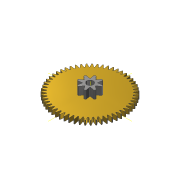
# Autodesk Inventor part: empty
Saved by Autodesk Inventor 2014 (Build 180170000, 170)
## iProperties
Created: 2015-04-13
Part Number: empty
Material: Generic
Document SubType Name: Modeling
Designer: Martin
Density: 1 g/cm^3
Appearance: Default
Author: Martin
Autodesk Inventor part; units mm, degrees
ref_plane "YZ Plane" through (0, 0, 0) normal (1, 0, 0) x (0, 1, 0)
ref_plane "XZ Plane" through (0, 0, 0) normal (0, 1, 0) x (-1, 0, 0)
ref_plane "XY Plane" through (0, 0, 0) normal (0, 0, 1) x (1, 0, 0)
sketch "Sketch1" plane through (0, 0, 0) normal (1, 0, 0) x (0, 1, 0)
  line L0 (0, -22.56081) -> (0, 23.084566)
  line L1 (-1.56, 0) -> (9.36, 0)
  line L2 (0, 16.563798) -> (0, -16.040042)
  line L3 (0.75, 0) -> (0.75, 2.8)
  line L4 (0.75, 2.8) -> (2.125, 2.8)
  line L5 (2.125, 2.8) -> (2.125, 1)
  line L6 (2.125, 1) -> (7.8, 1)
  line L7 (7.8, 1) -> (7.8, 0)
  line L8 (0.75, 0) -> (7.8, 0)
  point P0 (0, 0)
  dimension "d0" = 15.6
  dimension "d1" = 1
  dimension "d2" = 2.8
  dimension "d3" = 4.25
  dimension "d5" = 1.5
  constraints: 14 end point, 4 parallel, 4 point on line, 1 collinear, 1 perpendicular
  measures "d0" diameter of L7 L2
  measures "d1" distance of L6.end L7.end
  measures "d2" distance between parallel lines of L1 L4
  measures "d3" diameter of L5 L2
  measures "d5" diameter of L3 L2
sketch "Sketch1 outline for Revolution1" plane through (0, 0, 0) normal (1, 0, 0) x (0, 1, 0)
  line L0 (0.75, 2.8) -> (0.75, 0)
  line L1 (2.125, 2.8) -> (0.75, 2.8)
  line L2 (2.125, 1) -> (2.125, 2.8)
  line L3 (7.8, 1) -> (2.125, 1)
  line L4 (7.8, 0) -> (7.8, 1)
  line L5 (0.75, 0) -> (7.8, 0)
revolve "Revolution1" add sketch "Sketch1 outline for Revolution1" angle 360 about axis through (0, 0, 16.563798) along (0, 0, -1)
sketch "Sketch2" plane through (0, 0, 1) normal (0, 0, 1) x (1, 0, 0)
  circle A0 centre (0, 0) radius 2.125
  line L0 (0, -10.921041) -> (0, 10.926244)
  line L1 (0, 2.125) -> (0.44563, 7.78726) construction
  line L2 (0, 2.125) -> (-0.44563, 7.78726) construction
  line L3 (0, 6.646615) -> (-0.365996, 7.791409) construction
  line L4 (0, 6.646615) -> (0.365996, 7.791409) construction
  arc A1 (-0.095251, 6.944548) -> (0.095251, 6.944548) centre (0, 6.975) ccw
  line L5 (0, 6.975) -> (0, 7.8)
  circle A2 centre (0, 0) radius 7.8
  arc A3 (-0.342533, 7.71802) -> (-0.44563, 7.78726) centre (-0.437784, 7.687568) ccw
  arc A4 (0.44563, 7.78726) -> (0.342533, 7.71802) centre (0.437784, 7.687568) ccw
  line L6 (-0.095251, 6.944548) -> (-0.342533, 7.71802)
  line L7 (0.342533, 7.71802) -> (0.095251, 6.944548)
  dimension "d7" = 0.1
  dimension "d8" = 0.825
  dimension "d9" = 9
  dimension "d18" = 0.1
  constraints: 14 end point, 12 point on circle, 9 point on line, 8 tangent, 3 centre point, 2 collinear, 2 line through centre, 1 vertical alignment, 3 other
  measures "d7" radius of A1
  measures "d8" distance of L5.start L5.end
  measures "d9" angle of L1 L2
  measures "d18" radius of A3
sketch "Sketch2 outline for Extrusion4" plane through (0, 0, 1) normal (0, 0, 1) x (1, 0, 0)
  arc A0 (0.44563, 7.78726) -> (0.342533, 7.71802) centre (0.437784, 7.687568) ccw
  line L0 (0.342533, 7.71802) -> (0.095251, 6.944548)
  arc A1 (0.095251, 6.944548) -> (-0.095251, 6.944548) centre (0, 6.975) cw
  line L1 (-0.095251, 6.944548) -> (-0.342533, 7.71802)
  arc A2 (-0.342533, 7.71802) -> (-0.44563, 7.78726) centre (-0.437784, 7.687568) ccw
  arc A3 (0, 7.8) -> (-0.44563, 7.78726) centre (0, 0) ccw
  arc A4 (0.44563, 7.78726) -> (0, 7.8) centre (0, 0) ccw
extrude "Extrusion4" cut sketch "Sketch2 outline for Extrusion4" against normal through all
pattern_circular "Circular Pattern2" count 55 over 360 about axis through (0, 0, -10) along (0, 0, 1) of "Extrusion4"
sketch "Sketch3" plane through (0, 0, 2.8) normal (0, 0, 1) x (1, 0, 0)
  circle A0 centre (0, 0) radius 0.75
  circle A1 centre (0, 0) radius 2.125
  line L0 (0, -10.902595) -> (0, 10.902595)
  line L1 (0, 0.75) -> (-0.721066, 1.998922) construction
  line L2 (0, 0.75) -> (0.721066, 1.998922) construction
  line L3 (0, 1.125231) -> (-0.630709, 2.029244) construction
  line L4 (0, 1.125231) -> (0.630709, 2.029244) construction
  arc A2 (-0.082013, 1.242782) -> (0.082013, 1.242782) centre (0, 1.3) ccw
  line L5 (0, 1.3) -> (0, 2.125)
  arc A3 (-0.589053, 1.969538) -> (-0.721066, 1.998922) centre (-0.671066, 1.91232) ccw
  arc A4 (0.721066, 1.998922) -> (0.589053, 1.969538) centre (0.671066, 1.91232) ccw
  line L6 (-0.589053, 1.969538) -> (-0.082013, 1.242782)
  line L7 (0.082013, 1.242782) -> (0.589053, 1.969538)
  dimension "d28" = 0.825
  dimension "d29" = 0.1
  dimension "d30" = 60
  dimension "d31" = 0.1
  constraints: 14 end point, 13 point on circle, 8 tangent, 7 point on line, 3 centre point, 2 collinear, 2 line through centre, 2 other
  measures "d28" distance of L5.start L5.end
  measures "d29" radius of A2
  measures "d30" angle of L2 L1
  measures "d31" radius of A3
sketch "Sketch3 outline for Extrusion5" plane through (0, 0, 2.8) normal (0, 0, 1) x (1, 0, 0)
  arc A0 (0.686146, 2.011176) -> (0.589053, 1.969538) centre (0.671066, 1.91232) ccw
  line L0 (0.589053, 1.969538) -> (0.082013, 1.242782)
  arc A1 (0.082013, 1.242782) -> (-0.082013, 1.242782) centre (0, 1.3) cw
  line L1 (-0.082013, 1.242782) -> (-0.589053, 1.969538)
  arc A2 (-0.589053, 1.969538) -> (-0.686146, 2.011176) centre (-0.671066, 1.91232) ccw
  arc A3 (0, 2.125) -> (-0.686146, 2.011176) centre (0, 0) ccw
  arc A4 (0.686146, 2.011176) -> (0, 2.125) centre (0, 0) ccw
extrude "Extrusion5" cut sketch "Sketch3 outline for Extrusion5" against normal up to surface (1.8 mm away)
pattern_circular "Circular Pattern3" count 8 over 360 about axis through (0, 0, -10) along (0, 0, 1) of "Extrusion5"
body "Solid1"
